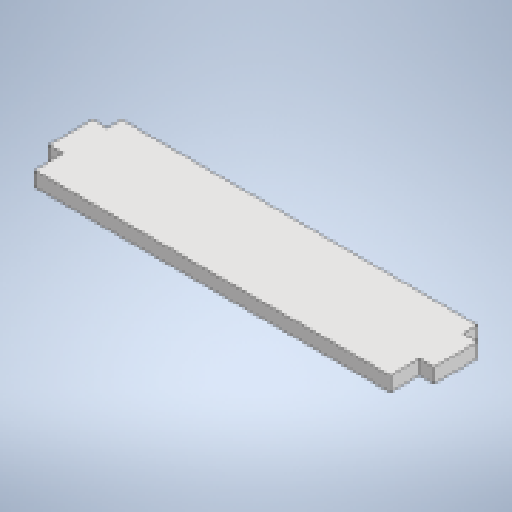
# Autodesk Inventor part: FANsuport
Saved by Autodesk Inventor 2023 (Build 270158000, 158)
## iProperties
Created: 2023-08-30
Part Number: FANsuport
Material: Generic
Document SubType Name: Modeling
Designer: Nathann
Density: 1 g/cm^3
Appearance: Default
Author: Nathann
Autodesk Inventor part; units mm, degrees
ref_plane "YZ Plane" through (0, 0, 0) normal (1, 0, 0) x (0, 1, 0)
ref_plane "XZ Plane" through (0, 0, 0) normal (0, 1, 0) x (-1, 0, 0)
ref_plane "XY Plane" through (0, 0, 0) normal (0, 0, 1) x (1, 0, 0)
sketch "Sketch1" plane through (0, 0, 0) normal (0, 0, 1) x (1, 0, 0)
  line L0 (0, 0) -> (-132, 0)
  line L1 (-132, 0) -> (-132, -5)
  line L2 (-132, -5) -> (0, -5)
  line L3 (0, -5) -> (0, 0)
  dimension "d0" = 5
  dimension "d1" = 132
  constraints: 8 end point, 2 parallel, 1 horizontal, 1 perpendicular
  measures "d0" distance between parallel lines of L0 L2
  measures "d1" distance of L1.end L2.end
extrude "Extrusion1" add sketch "Sketch1" along normal blind 30
sketch "Sketch2" plane through (-132, 0, 0) normal (0, 1, 0) x (1, 0, 0)
  line L0 (0, -30) -> (132, -30) projected
  line L1 (0, -30) -> (5, -30)
  line L2 (5, -30) -> (5, -15)
  line L3 (5, -15) -> (0, -15)
  line L4 (0, -15) -> (0, -30)
  line L5 (132, -30) -> (127, -30)
  line L6 (127, -30) -> (127, -15)
  line L7 (127, -15) -> (132, -15)
  line L8 (132, -15) -> (132, -30)
  line L9 (0, 0) -> (0, -30) projected
  line L10 (132, 0) -> (132, -30) projected
  line L11 (0, 0) -> (132, 0)
  line L12 (132, 0) -> (132, 0)
  line L13 (132, 0) -> (0, 0)
  line L14 (0, 0) -> (0, 0)
  line L15 (0, 0) -> (5, 0)
  line L16 (5, 0) -> (5, -5)
  line L17 (5, -5) -> (0, -5)
  line L18 (0, -5) -> (0, 0)
  line L19 (132, 0) -> (127, 0)
  line L20 (127, 0) -> (127, -5)
  line L21 (127, -5) -> (132, -5)
  line L22 (132, -5) -> (132, 0)
  point P0 (5, -30)
  point P1 (5, 0)
  point P2 (127, 0)
  dimension "d4" = 5
  dimension "d5" = 15
  dimension "d6" = 15
  dimension "d7" = 5
  dimension "d8" = 0
  dimension "d11" = 5
  dimension "d12" = 5
  dimension "d13" = 5
  dimension "d14" = 10
  constraints: 40 end point, 10 equal length, 5 horizontal, 5 perpendicular, 1 point on line
  measures "d4" distance of L2.end L3.end
  measures "d5" distance of L3.end L0.start
  measures "d6" distance of L7.end L0.end
  measures "d7" distance of L6.end L7.end
  measures "d8" distance between parallel lines of L11 L13
  measures "d11" distance of L16.end L17.end
  measures "d12" distance of L15.end L16.end
  measures "d13" distance of L19.end L20.end
  measures "d14" distance between parallel lines of L21 L7
extrude "Extrusion2" cut sketch "Sketch2" against normal blind 10 contours L4 L3 L2 L0 | L6 L7 L8 L0 | L9 L11 L16 L17 | L21 L20 L11 L10
body "Solid1"
